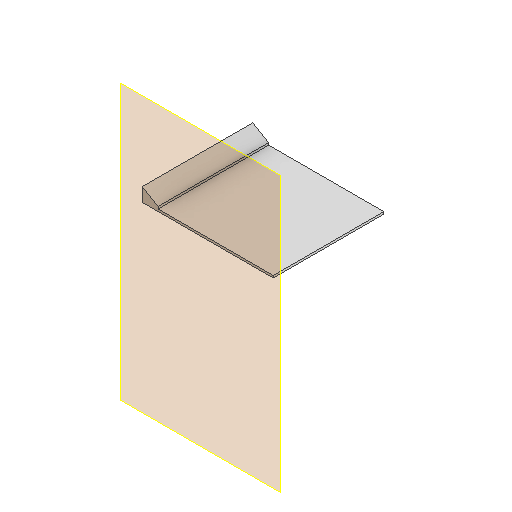
# Autodesk Inventor part: IM_ledmatrix_diffuser
Saved by Autodesk Inventor 2022 (Build 260153000, 153)
## iProperties
Created: 2023-06-20
Part Number: IM_ledmatrix_diffuser
Material: Generisch
Document SubType Name: Modeling
Designer: diederichbenedict
Density: 1 g/cm^3
Appearance: Vorgabe
Author: diederichbenedict
Autodesk Inventor part; units mm, degrees
ref_plane "YZ Plane" through (0, 0, 0) normal (1, 0, 0) x (0, 1, 0)
ref_plane "XZ Plane" through (0, 0, 0) normal (0, 1, 0) x (-1, 0, 0)
ref_plane "Arbeitsebene1" through (0, 0, 0) normal (0, 0, 1) x (1, 0, 0)
sketch "Skizze1" plane through (0, 0, 0) normal (0, 0, 1) x (1, 0, 0)
  line L0 (3, 37.7407) -> (3, 42.1841) projected
  line L1 (3, 42.1841) -> (4.4798, 41.3297) projected
  line L2 (4.4798, 41.3297) -> (4.4798, 50) projected
  line L3 (3.1236, 50) -> (4.4798, 50) projected
  line L4 (3.1236, 50) -> (3.1236, 54) projected
  line L5 (3.1236, 54) -> (33.1034, 54) projected
  line L6 (33.1034, 54) -> (33.1034, 58) projected
  line L7 (-0.0202, 58) -> (33.1034, 58) projected
  line L8 (-0.0202, 20) -> (-0.0202, 58) projected
  line L9 (4.4798, 20) -> (4.4798, 37.7407) projected
  line L10 (4.5, 37.1634) -> (4.7348, 37.2989) projected
  line L11 (4.4798, 37.7407) -> (6.4798, 37.7407) projected
  line L12 (6.4798, 40.7407) -> (5.5, 40.7407) projected
  line L13 (5.5, 40.7407) -> (4.4798, 41.3297) projected
  line L14 (4.4, 41.1449) -> (3.2, 41.8377)
  line L15 (3.2, 41.8377) -> (3.2, 36.6437)
  line L16 (3.2, 36.6437) -> (4.4, 37.3366)
  line L17 (4.4, 41.1449) -> (6.8321, 39.7407)
  line L18 (6.8321, 39.7407) -> (6.8321, 38.7407)
  line L19 (6.8321, 38.7407) -> (4.4, 37.3366)
  line L20 (33.1236, 40.3183) -> (33.1236, 39.2407)
  line L21 (33.1236, 39.2407) -> (6.8321, 39.2407)
  line L22 (33.1236, 39.2407) -> (6.8321, 39.2407)
  line L23 (6.8321, 39.2407) -> (6.8321, 38.7407)
  line L24 (6.8321, 38.7407) -> (33.1236, 38.7407)
  line L25 (33.1236, 38.7407) -> (33.1236, 39.2407)
  line L26 (6.8321, 38.7407) -> (3.2, 38.7407)
  line L27 (-0.0202, 20) -> (4.4798, 20) projected
  line L28 (4.4798, 37.7407) -> (3, 37.7407) projected
  point P0 (4.5, 37.1634)
  dimension "d0" = 0.2
  dimension "d3" = 0.5
  dimension "d4" = 1.4042
  constraints: 26 end point, 2 parallel, 2 perpendicular, 2 point on line, 1 horizontal, 1 midpoint, 1 vertical, 2 other
  measures "d0" distance between parallel lines of L1 L14
  measures "d3" distance between parallel lines of L24 L21
  measures "d4" vertical distance of L18.end L19.end
ref_plane "Arbeitsebene2" through (-0.0423, 0, -25.2444) normal (0, 0, -1) x (0, 1, 0)
extrude "Extrusion1" add sketch "Skizze1" against normal up to surface (25.2444 mm away) contours L15 L14 L17 L18 L26 | L18 L21 L25 L24
